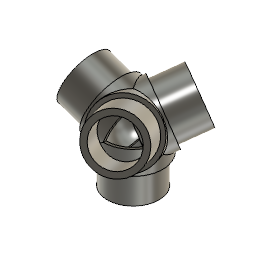
node-no-legs-not-rounded (Autodesk Fusion 360 design; units mm, degrees)
Autodesk Fusion 360 part; units mm, degrees
sketch "Skizze1" plane through (0, 0, 0) normal (0, 0, 1) x (1, 0, 0)
  circle A0 centre (0, 0) radius 23
  circle A1 centre (0, 0) radius 20
  circle A2 centre (0, 0) radius 15.75
extrude "Extrusion1" add sketch "Skizze1" against normal blind 18 contours A0 makes body 1
extrude "Extrusion2" add sketch "Skizze1" against normal blind 40 separate body contours A1 makes body 2
combine "Kombinieren1" operation add target body 1 tool bodies 2
sketch "Skizze2" plane through (0, 0, 0) normal (0, 0, 1) x (1, 0, 0)
  circle A0 centre (0, 0) radius 23
  circle A1 centre (0, 0) radius 20
  circle A2 centre (0, 0) radius 15.75
extrude "Extrusion3" add sketch "Skizze2" against normal blind 18 separate body contours A0 makes body 3
extrude "Extrusion4" add sketch "Skizze2" against normal blind 40 separate body contours A1 makes body 4
combine "Kombinieren2" operation add target body 3 tool bodies 4
move_body "Verschieben1" bodies 3 to x (-0.333333, 0, -0.942809) y (0, 1, 0) z (0.942809, 0, -0.333333) at (0, 0, 0)
pattern_circular "C-Anordnung1" count 3 over 360 about axis through (0, 0, 1.75) along (0, 0, 1) of bodies 3 makes body 5 at (15.8724, -25.9217, -5.9419) makes body 6 at (7.5393, 16.1948, -10.331)
combine "Kombinieren3" operation add target body 1 tool bodies 3 5 6
sketch "Skizze3" plane through (0, 0, 0) normal (0, 0, 1) x (1, 0, 0)
  arc A0 (0, 21) -> (0, -21) centre (0, 0) ccw
  line L0 (0, 21) -> (0, -21)
revolve "Drehen1" cut sketch "Skizze3" angle 360 about axis through (0, 1.75, 0) along (0, 1, 0) bodies 1
equation "arm_outer_diameter = 46 mm" comment "Aussendurchmesser aller 4 Arme"
equation "arm_depth = 40 mm" comment "Armlaenge gemessen vom Zentrum"
equation "ring_inner_diameter = 40 mm" comment "Durchmesser der erhabenen Stirnflaeche"
equation "ring_extrude_depth = 22 mm" comment "Tiefe des Rumpfabsatzes / Rücksprungs"
equation "hole_diameter = 31.5 mm" comment "Durchmesser der zentrischen Bohrung"
equation "inner_ball_diameter = 42 mm" comment "Durchmesser des inneren Kugelloches"
equation "d7 = -arm_depth + ring_extrude_depth"
equation "d9 = -arm_depth"
equation "d11 = -arm_depth + ring_extrude_depth"
equation "d13 = -arm_depth"
named bodies: "Node"
